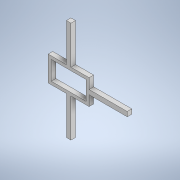
# Autodesk Inventor part: FS90R-Foot
Saved by Autodesk Inventor 2022 (Build 260153000, 153)
## iProperties
Created: 2024-06-18
Part Number: FS90R-Foot
Material: 一般
Document SubType Name: Modeling
Designer: yamashita1
Density: 1 g/cm^3
Appearance: 既定
Author: yamashita1
Autodesk Inventor part; units mm, degrees
ref_plane "YZ Plane" through (0, 0, 0) normal (1, 0, 0) x (0, 1, 0)
ref_plane "XZ Plane" through (0, 0, 0) normal (0, 1, 0) x (-1, 0, 0)
ref_plane "XY Plane" through (0, 0, 0) normal (0, 0, 1) x (1, 0, 0)
derived "FS90R.ipt"
sketch "スケッチ2" plane through (0, 0, 0) normal (0, 0, 1) x (1, 0, 0)
  line L0 (-11.4, 6.2) -> (11.4, 6.2)
  line L1 (11.4, 6.2) -> (11.4, -6.2)
  line L2 (11.4, -6.2) -> (-11.4, -6.2)
  line L3 (-11.4, -6.2) -> (-11.4, 6.2)
  line L4 (-13.4, 8.2) -> (13.4, 8.2)
  line L5 (13.4, 8.2) -> (13.4, -8.2)
  line L6 (13.4, -8.2) -> (-13.4, -8.2)
  line L7 (-13.4, -8.2) -> (-13.4, 8.2)
  line L8 (13.4, 1.5) -> (38.4, 1.5)
  line L9 (38.4, 1.5) -> (38.4, -1.5)
  line L10 (38.4, -1.5) -> (13.4, -1.5)
  line L11 (13.4, -1.5) -> (13.4, 1.5)
  line L12 (-1.5, 8.2) -> (1.5, 8.2)
  line L13 (1.5, 8.2) -> (1.5, 33.2)
  line L14 (1.5, 33.2) -> (-1.5, 33.2)
  line L15 (-1.5, 33.2) -> (-1.5, 8.2)
  line L16 (-1.5, -8.2) -> (1.5, -8.2)
  line L17 (1.5, -8.2) -> (1.5, -33.2)
  line L18 (1.5, -33.2) -> (-1.5, -33.2)
  line L19 (-1.5, -33.2) -> (-1.5, -8.2)
  point P0 (0, 0)
  point P1 (11.4, 0)
  point P2 (0, 6.2)
  point P3 (-13.4, 0)
  point P4 (0, -8.2)
  point P5 (13.4, 0)
  point P6 (0, 8.2)
  point P7 (0, -8.2)
  point P8 (13.4, -1.5)
  dimension "d1" = 12.4
  dimension "d2" = 22.8
  dimension "WAKU" = 2
  dimension "d4" = 2
  dimension "FOOT_LEN" = 25
  dimension "FOOT_WIDTH" = 3
  constraints: 40 end point, 10 parallel, 9 perpendicular, 7 midpoint, 5 horizontal, 4 vertical alignment, 3 horizontal alignment, 3 point on line
  measures "d1" distance of L0.end L1.end
  measures "d2" distance of L0.start L0.end
  measures "WAKU" distance between parallel lines of L7 L3
  measures "d4" distance between parallel lines of L6 L2
  measures "FOOT_LEN" distance of L9.end L10.end
  measures "FOOT_WIDTH" distance of L8.end L9.end
extrude "押し出し1" add sketch "スケッチ2" along normal blind 3
equation "\"d4\" = WAKU"
